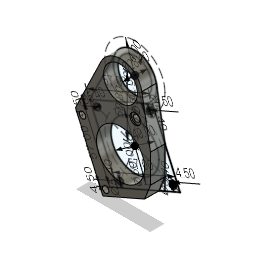
stepper-mount-nema23-28mm-hole (Autodesk Fusion 360 design; units mm, degrees)
Autodesk Fusion 360 part; units mm, degrees
sketch "Sketch1" plane through (0, 0, 0) normal (0, 0, 1) x (1, 0, 0)
  circle A0 centre (0, 0) radius 14.05
  circle A1 centre (0, 0) radius 18.05
  line L0 (0, 0) -> (0, -50.8) construction
  line L1 (14.7041, -13.2728) -> (-37.5272, -36.0959)
  line L2 (-37.5272, -36.0959) -> (-14.7041, -88.3272)
  line L3 (-14.7041, -88.3272) -> (37.5272, -65.5041)
  line L4 (37.5272, -65.5041) -> (14.7041, -13.2728)
  line L5 (-37.5272, -36.0959) -> (37.5272, -65.5041) construction
  line L6 (14.7041, -13.2728) -> (-14.7041, -88.3272) construction
  circle A2 centre (0, -50.8) radius 25 construction
  line L7 (25, -36.8353) -> (25, -70.978)
  circle A3 centre (0, -50.8) radius 20
  circle A4 centre (12.3824, -19.1982) radius 2.7
  circle A5 centre (-31.6018, -38.4176) radius 2.7
  circle A6 centre (-12.3824, -82.4018) radius 2.7
  circle A7 centre (31.6018, -63.1824) radius 2.7
  line L8 (25, -36.8353) -> (17.7622, 3.2103)
  line L9 (-37.5272, -36.0959) -> (-16.2465, 7.8647)
  circle A8 centre (0, 0) radius 25 construction
  circle A9 centre (12.3824, -19.1982) radius 4.5
  line L10 (25, -60.5957) -> (20.0915, -73.1228)
  point P0 (0, -50.8)
  dimension "d1" = 28.1
  dimension "d2" = 4
  dimension "d3" = 50.8
  dimension "d4" = 57
  dimension "d5" = 57
  dimension "d6" = 57
  dimension "d7" = 50
  dimension "d8" = 40
  dimension "d9" = 5.4
  dimension "d10" = 4.5
  dimension "d11" = 5.4
  dimension "d12" = 5.4
  dimension "d13" = 5.4
  dimension "d14" = 4.5
  dimension "d15" = 4.5
  dimension "d16" = 4.5
  dimension "d19" = 50
  constraint coincident A0.centre A1.centre
  constraint vertical L0
  constraint perpendicular L1 L2
  constraint perpendicular L2 L3
  constraint midpoint L5 P0
  constraint coincident P0 L0.end
  constraint tangent A1 L1
  constraint coincident L4 L7.start
  constraint coincident L3 L7.end
  constraint vertical L7
  constraint tangent A2 L7
  constraint coincident L6 A4.centre
  constraint coincident L5 A5.centre
  constraint coincident L6 A6.centre
  constraint coincident L5 A7.centre
  constraint coincident A1 L8.end
  constraint tangent A1 L8
  constraint coincident A1 L9.end
  constraint tangent A1 L9
  constraint concentric A4 A9
  constraint tangent L1 A9
  constraint coincident L7 L10.start
  constraint coincident L5 L10.start
  constraint coincident L3 L10.end
  constraint perpendicular L5 L10
  measures "d1" diameter of A0
  measures "d3" distance of A0.centre P0
  measures "d4" distance of L1.start L1.end
  measures "d5" distance of L1.end L2.end
  measures "d6" distance of L2.end L3.end
  measures "d7" diameter of A2
  measures "d8" diameter of A3
  measures "d9" diameter of A4
  measures "d10" distance of L4 A4.centre
  measures "d11" diameter of A5
  measures "d12" diameter of A6
  measures "d13" diameter of A7
  measures "d14" distance of L4 A7.centre
  measures "d15" distance of L3 A6.centre
  measures "d16" distance of L1 A5.centre
  measures "d19" diameter of A8
extrude "Extrude1" add sketch "Sketch1" along normal blind 12 contours A1 | A1 L1 L4 L8 | A1 L1 L9 | L1 L2 L3 L4 L7 A9 L10 | L1 L4 A9 | A9 | L3 L7 L10
extrude "Extrude2" cut sketch "Sketch1" along normal blind 1 from surface at 11 contours A9
extrude "Extrude3" cut sketch "Sketch1" along normal blind 12 contours L3 L7 L10
